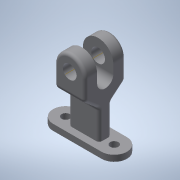
# Autodesk Inventor part: Fitting
Saved by Autodesk Inventor 2020 (Build 240168000, 168)
## iProperties
Created: 2021-11-30
Part Number: Fitting
Material: Generic
Document SubType Name: Modeling
Designer: Manuel
Density: 1 g/cm^3
Appearance: Default
Author: Manuel
Autodesk Inventor part; units mm, degrees
ref_plane "YZ Plane" through (0, 0, 0) normal (1, 0, 0) x (0, 1, 0)
ref_plane "XZ Plane" through (0, 0, 0) normal (0, 1, 0) x (-1, 0, 0)
ref_plane "XY Plane" through (0, 0, 0) normal (0, 0, 1) x (1, 0, 0)
sketch "Sketch1" plane through (0, 0, 0) normal (0, 1, 0) x (-1, 0, 0)
  arc A0 (15, 60) -> (-15, 60) centre (0, 60) ccw
  line L0 (-15, 60) -> (-15, 0)
  line L1 (-15, 0) -> (15, 0)
  line L2 (15, 0) -> (15, 60)
  line L3 (21, 0) -> (-21, 0) projected
  line L4 (0, -15) -> (0, 90) projected
  circle A1 centre (0, 60) radius 6.7766
  point P0 (0, 0)
  dimension "d0" = 30
  dimension "d1" = 60
  dimension "d2" = 15
  constraints: 6 end point, 2 centre point, 2 parallel, 2 point on circle, 1 coincident, 1 horizontal, 1 midpoint, 1 point on line, 1 vertical
  measures "d0" distance between parallel lines of L0 L2
  measures "d1" distance from line of A0.centre L1
  measures "d2" radius of A0
extrude "Extrusion1" add sketch "Sketch1" along normal mid plane 40 contours L2 L1 L4 A1 A0 | L4 A1 L1 L0 A0
sketch "Sketch2" plane through (15, -20, 0) normal (1, 0, 0) x (0, 0, -1)
  line L0 (0, 0) -> (0, 40) projected
  line L1 (-60, 40) -> (0, 40) projected
  line L2 (0, 0) -> (-60, 0) projected
  line L3 (-60, 40) -> (-60, 40) projected
  line L4 (-60, 0) -> (-60, 0) projected
  line L5 (-75, 0) -> (-75, 40) projected
  line L6 (-75, 12) -> (-51.3579, 12)
  line L7 (-51.3579, 28) -> (-75, 28)
  line L8 (-75, 28) -> (-75, 12)
  line L9 (-53.2234, 0) -> (-66.7766, 0) projected
  line L10 (-93.6547, 20) -> (5.2074, 20) construction
  line L11 (-40.607, 0) -> (-28.8596, 14)
  line L12 (-28.8596, 14) -> (0, 14)
  line L13 (0, 0) -> (0, 40) construction
  line L14 (-40.607, 40) -> (-28.8596, 26)
  line L15 (-28.8596, 26) -> (0, 26)
  line L16 (0, 0) -> (-60, 0) construction
  line L17 (-60, 40) -> (0, 40) construction
  arc A0 (-51.3579, 12) -> (-51.3579, 28) centre (-51.3579, 20) ccw
  line L18 (-53.2234, 0) -> (-66.7766, 0) projected
  line L19 (-66.7766, 40) -> (-53.2234, 40) projected
  line L20 (-53.2234, 40) -> (-53.2234, 0) projected
  point P0 (0, 20)
  point P1 (-75, 20)
  point P2 (0, 20)
  point P3 (-40.607, 0)
  dimension "d5" = 130
  dimension "d6" = 12
  dimension "d7" = 16
  dimension "d8" = 8
  constraints: 16 end point, 7 point on line, 3 parallel, 2 horizontal, 2 midpoint, 2 perpendicular, 2 point on circle, 1 centre point, 1 vertical, 1 other
  measures "d5" angle of L12 L11
  measures "d6" distance between parallel lines of L15 L12
  measures "d7" distance of L7.end L6.start
  measures "d8" radius of A0
extrude "Extrusion2" cut sketch "Sketch2" against normal blind 40 contours L2 L11 L12 L0 | L15 L14 L1 L0 | L20 L7 A0 L6 | L6 L5 L7 L20
fillet "Fillet1" radius 5 4 edges at (0, -20, 40.607) (0, -6, 28.8596) (0, 6, 28.8596) (0, 20, 40.607)
fillet "Fillet2" radius 3 22 edges at (-15, -20, 51.4693) (-15, -19.5315, 40.8254) (-15, -13, 34.7333) (-15, -6.4685, 28.6411) (-15, -6, 13.264) (15, -20, 51.4693) (15, -19.5315, 40.8254) (15, -13, 34.7333) (15, -6.4685, 28.6411) (15, -6, 13.264) (0, -20, 75) (15, 20, 51.4693) (15, 19.5315, 40.8254) (15, 13, 34.7333) (15, 6.4685, 28.6411) (15, 6, 13.264) (-15, 20, 51.4693) (-15, 19.5315, 40.8254) (-15, 13, 34.7333) (-15, 6.4685, 28.6411) (-15, 6, 13.264) (0, 20, 75)
sketch "Sketch3" plane through (12, -6, 0) normal (0, 0, -1) x (-1, 0, 0)
  arc A0 (0, 12) -> (-3, 9) centre (0, 9) ccw projected
  line L0 (-3, 3) -> (-3, 9) projected
  arc A1 (-3, 3) -> (0, 0) centre (0, 3) ccw projected
  line L1 (0, 0) -> (24, 0) projected
  arc A2 (24, 0) -> (27, 3) centre (24, 3) ccw projected
  line L2 (27, 9) -> (27, 3) projected
  arc A3 (27, 9) -> (24, 12) centre (24, 9) ccw projected
  line L3 (24, 12) -> (0, 12) projected
  line L4 (-11.8816, 6) -> (35.8816, 6) construction
  line L5 (-11.8816, -6.5) -> (35.8816, -6.5)
  line L6 (35.8816, 18.5) -> (-11.8816, 18.5)
  arc A4 (-11.8816, 18.5) -> (-11.8816, -6.5) centre (-11.8816, 6) ccw
  arc A5 (35.8816, -6.5) -> (35.8816, 18.5) centre (35.8816, 6) ccw
  circle A6 centre (35.8816, 6) radius 4.0304
  circle A7 centre (-11.8816, 6) radius 4.0304
  point P0 (12, 6)
  point P1 (12, 6)
  dimension "d13" = 25
  constraints: 8 end point, 4 centre point, 4 point on circle, 4 tangent, 3 coincident, 1 equal radius, 1 horizontal, 1 midpoint, 1 parallel
  measures "d13" distance between parallel lines of L6 L5
extrude "Extrusion3" add sketch "Sketch3" along normal blind 6 contours L3 A3 L2 A2 L1 A1 L0 A0 | A4 L6 A5 L5
body "Solid1"
